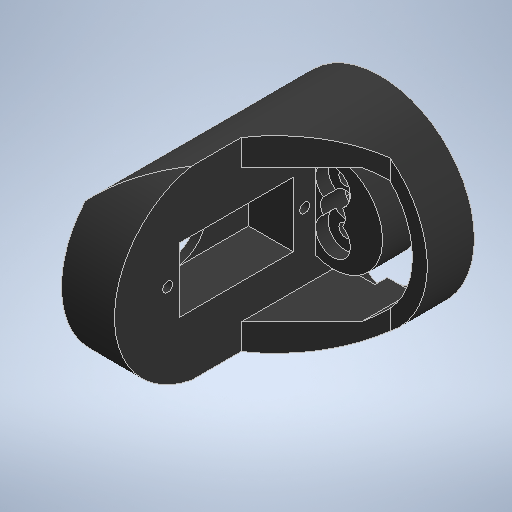
# Autodesk Inventor part: BracoRobotico_0007_001
Saved by Autodesk Inventor 2025.2 (Build 292293000, 293)
## iProperties
Created: 2025-05-22
Part Number: BracoRobotico_0007_001
Material: Rubber
Document SubType Name: Modeling
Designer: I
Density: 0.93 g/cm^3
Appearance: Rubber - Black
Author: I
Autodesk Inventor part; units mm, degrees
sketch "Sketch30" plane through (0, 0, 0) normal (0, 0, 1) x (1, 0, 0)
  circle A0 centre (0, 0) radius 19
  dimension "d252" = 38
  constraints: 1 centre point, 1 coincident
  measures "d252" diameter of A0
extrude "Extrusion28" add sketch "Sketch30" along normal mid plane 50
sketch "Sketch33" plane through (0, 0, 0) normal (0, 1, 0) x (-1, 0, 0)
  line L0 (19, -15.5) -> (14.2, -15.5)
  line L1 (14.2, -15.5) -> (14.2, 25)
  line L2 (14.2, 25) -> (19, 25)
  line L3 (19, 25) -> (19, -15.5)
  line L4 (19, -15.5) -> (14.2, 25) construction
  line L5 (14.2, -15.5) -> (19, 25) construction
  line L6 (19, 25) -> (-19, 25) construction
  line L7 (3.5, -15.5) -> (-19, -15.5)
  line L8 (-19, -15.5) -> (-19, 25)
  line L9 (-19, 25) -> (3.5, 25)
  line L10 (3.5, 25) -> (3.5, -15.5)
  line L11 (3.5, -15.5) -> (-19, 25) construction
  line L12 (-19, -15.5) -> (3.5, 25) construction
  point P0 (0, 0)
  point P1 (16.6, 4.75)
  point P2 (-7.75, 4.75)
  dimension "d253" = 14.2
  dimension "d254" = 40.5
  dimension "d277" = 10.7
  constraints: 24 end point, 4 midpoint, 2 perpendicular, 1 horizontal, 1 parallel
  measures "d253" distance from line of point (0, 0) L1
  measures "d254" distance of L2.end L0.start
  measures "d277" distance between parallel lines of L1 L10
extrude "Extrusion34" cut sketch "Sketch33" along normal mid plane 50
sketch "Sketch35" plane through (0, 0, 0) normal (1, 0, 0) x (0, 1, 0)
  circle A0 centre (0, 6) radius 19
  line L0 (0, 25) -> (-28, 25)
  line L1 (-28, 25) -> (-19, 6)
  line L2 (0, 6) -> (-19, 6) construction
  line L3 (28, 25) -> (19, 6)
  line L4 (-18.6748, 25) -> (18.6748, 25) projected
  line L5 (0, 25) -> (28, 25)
  point P0 (0, 0)
  dimension "d257" = 38
  dimension "d258" = 28
  constraints: 10 end point, 3 horizontal, 3 point on circle, 1 centre point, 1 coincident, 1 collinear, 1 horizontal alignment, 1 midpoint, 1 tangent, 1 vertical alignment
  measures "d257" diameter of A0
  measures "d258" distance of L0.start L0.end
extrude "Extrusion35" cut sketch "Sketch35" along normal through all both and the other way through all contours A0 L4 L5 L3 | A0 L1 L0
sketch "Sketch36" plane through (-14.2, -12.6238, -15.5) normal (-1, 0, 0) x (0, 0, 1)
  circle A0 centre (19.5, 12.6238) radius 6.5 construction
  line L0 (19.5, 19.1238) -> (19.5, 6.1238) construction
  line L1 (19.5, 19.1238) -> (27.5, 19.1238)
  line L2 (27.5, 19.1238) -> (27.5, 6.1238)
  line L3 (27.5, 6.1238) -> (19.5, 6.1238)
  arc A1 (19.5, 19.1238) -> (19.5, 6.1238) centre (19.5, 12.6238) ccw
  arc A2 (35.7, 0) -> (35.7, 25.2476) centre (21.5, 12.6238) ccw construction
  arc A3 (25, -6.0511) -> (35.7, 0) centre (21.5, 12.6238) ccw construction
  arc A4 (35.7, 25.2476) -> (25, 31.2986) centre (21.5, 12.6238) ccw construction
  line L4 (27.5, 19.1238) -> (34, 12.6238)
  line L5 (34, 12.6238) -> (27.5, 6.1238)
  line L6 (27.5, 12.6238) -> (34, 12.6238) construction
  circle A5 centre (30.5, 12.6238) radius 1
  arc A6 (25, -6.0511) -> (25, 31.2986) centre (21.5, 12.6238) ccw construction
  point P0 (15.5, 12.6238)
  dimension "d261" = 13
  dimension "d262" = 8
  dimension "d265" = 6.5
  dimension "d271" = 2
  dimension "d272" = 9
  dimension "d278" = 2
  constraints: 14 end point, 3 perpendicular, 2 centre point, 2 coincident, 2 midpoint, 2 point on circle, 1 horizontal, 1 horizontal alignment, 1 point on line, 1 vertical, 1 vertical alignment, 2 other
  measures "d262" distance of L0.start L1.end
  measures "d265" distance of L6.start L4.end
  measures "d271" diameter of A5
  measures "d272" distance of A3.centre A5.centre
  measures "d278" distance of A3.centre point (19.5, 12.624)
extrude "Extrusion36" cut sketch "Sketch36" along normal through all both and the other way through all contours L1 L2 L3 A1
extrude "Extrusion37" cut sketch "Sketch36" against normal blind 2 contours L4 L5 L2 | A5
sketch "Sketch38" plane through (-3.5, -18.6748, -15.5) normal (1, 0, 0) x (0, 0, -1)
  line L0 (-4.5, 12.1748) -> (-27.5, 12.1748)
  line L1 (-27.5, 12.1748) -> (-27.5, 25.1748)
  line L2 (-27.5, 25.1748) -> (-4.5, 25.1748)
  line L3 (-4.5, 25.1748) -> (-4.5, 12.1748)
  line L4 (-4.5, 12.1748) -> (-27.5, 25.1748) construction
  line L5 (-27.5, 12.1748) -> (-4.5, 25.1748) construction
  circle A0 centre (-29.8, 18.6748) radius 1
  circle A1 centre (-2.2, 18.6748) radius 1
  point P0 (-15.5, 18.6748)
  point P1 (-16, 18.6748)
  dimension "d281" = 23
  dimension "d282" = 13
  dimension "d286" = 2
  dimension "d287" = 2.3
  dimension "d288" = 2.3
  dimension "d289" = 2
  constraints: 12 end point, 3 horizontal alignment, 2 centre point, 2 midpoint, 1 perpendicular
  measures "d281" distance of L1.end L2.end
  measures "d282" distance of L1.end L0.end
  measures "d286" diameter of A0
  measures "d287" distance from line of L1 A0.centre
  measures "d288" distance from line of L3 A1.centre
  measures "d289" diameter of A1
extrude "Extrusion40" cut sketch "Sketch38" against normal blind 9 contours L0 L1 L2 L3
extrude "Extrusion41" cut sketch "Sketch38" along normal through all both and the other way through all contours A0 | A1
sketch "Sketch39" plane through (0, 0, -25) normal (0, 0, -1) x (-1, 0, 0)
  circle A0 centre (0, 0) radius 16
  dimension "d292" = 32
  constraints: 1 centre point, 1 coincident
  measures "d292" diameter of A0
extrude "Extrusion42" cut sketch "Sketch39" against normal blind 2
sketch "Sketch40" plane through (0, 0, -23) normal (0, 0, -1) x (-1, 0, 0)
  circle A0 centre (0, 0) radius 10
  line L0 (3.5, -9.3675) -> (3.5, -13.5)
  line L1 (3.5, -13.5) -> (-8.5878, -13.5)
  line L2 (3.5, 9.3675) -> (3.5, 13.5)
  line L3 (3.5, 13.5) -> (-8.5878, 13.5)
  circle A1 centre (0, 0) radius 16 construction
  arc A2 (-8.5878, 13.5) -> (-8.5878, -13.5) centre (0, 0) ccw
  dimension "d295" = 20
  dimension "d296" = 3.5
  dimension "d297" = 27
  constraints: 8 end point, 6 point on circle, 2 centre point, 2 coincident, 2 equal length, 2 horizontal, 1 collinear
  measures "d295" diameter of A0
  measures "d296" distance from line of point (0, 0) L0
  measures "d297" distance between parallel lines of L3 L1
extrude "Extrusion43" cut sketch "Sketch40" along normal through all both and the other way through all contours A0 L0 L1 A2 L3 L2
sketch "Sketch41" plane through (0, 0, -25) normal (0, 0, -1) x (-1, 0, 0)
  circle A0 centre (0, -14) radius 3.5
  line L0 (0, -14) -> (0, 0) construction
  dimension "d300" = 7
  dimension "d301" = 14
  constraints: 2 end point, 1 centre point, 1 vertical
  measures "d300" diameter of A0
  measures "d301" distance of L0.end L0.start
extrude "Extrusion44" cut sketch "Sketch41" against normal blind 4.5
mirror "Mirror2" about plane through (0, 0, 0) normal (0, 1, 0) of "Extrusion44"
sketch "Sketch42" plane through (0, 0, -23) normal (0, 0, -1) x (-1, 0, 0)
  circle A0 centre (0, 0) radius 5 construction
  line L0 (0, -10) -> (0, 0) construction
  arc A1 (3.5, 9.3675) -> (3.5, -9.3675) centre (0, 0) ccw construction
  arc A2 (-3.75, -9.2702) -> (3.75, -9.2702) centre (0, 0) ccw
  line L1 (-4.1758, -2.75) -> (-4.1758, 2.75) construction
  line L2 (-4.1758, -2.75) -> (-3.75, -9.2702)
  arc A3 (-4.1758, 2.75) -> (-4.1758, -2.75) centre (0, 0) ccw
  line L3 (-4.1758, 2.75) -> (-3.75, 9.2702)
  line L4 (0, 10) -> (0, -10)
  arc A4 (0, 10) -> (-3.75, 9.2702) centre (0, 0) ccw
  point P0 (-4.1758, 0)
  dimension "d305" = 10
  dimension "d306" = 7.5
  dimension "d307" = 5.5
  constraints: 13 point on circle, 10 end point, 4 centre point, 4 coincident, 3 vertical, 2 midpoint, 1 concentric, 1 equal length, 1 horizontal alignment, 1 point on line
  measures "d305" diameter of A0
  measures "d306" distance of A2.end L2.end
  measures "d307" distance of L1.start L1.end
extrude "Extrusion45" cut sketch "Sketch42" against normal blind 2.5
mirror "Mirror3" about plane through (0, 0, 0) normal (1, 0, 0) of "Extrusion45"
sketch "Sketch43" plane through (0, 0, -20.5) normal (0, 0, -1) x (-1, 0, 0)
  circle A0 centre (0, 0) radius 2.5
  circle A1 centre (0, 4.5) radius 1.3
  circle A2 centre (0, -4.5) radius 1.3
  line L0 (0, -4.5) -> (0, 4.5) construction
  dimension "d310" = 5
  dimension "d311" = 2.6
  dimension "d312" = 9
  constraints: 4 coincident, 3 centre point, 2 end point, 1 equal radius, 1 midpoint, 1 vertical
  measures "d310" diameter of A0
  measures "d311" diameter of A2
  measures "d312" distance of L0.start L0.end
extrude "Extrusion46" cut sketch "Sketch43" against normal up to surface (5 mm away)
chamfer "Chamfer4" distance 15 angle 45 2 edges at (-3.5, -16.0874, -15.5) (-3.5, 16.0874, -15.5)
sketch "Sketch44" plane through (0, 0, -15.5) normal (0, 0, 1) x (1, 0, 0)
  circle A0 centre (0, -4.5) radius 1.3 projected
  circle A1 centre (0, 4.5) radius 1.3 projected
  circle A2 centre (0, 4.5) radius 3.5
  circle A3 centre (0, -4.5) radius 3.5
  point P0 (0, 0)
  dimension "d318" = 7
  constraints: 2 centre point, 2 coincident, 1 equal radius
  measures "d318" diameter of A2
extrude "Extrusion47" cut sketch "Sketch44" against normal blind 2.5
body "Solid3"
